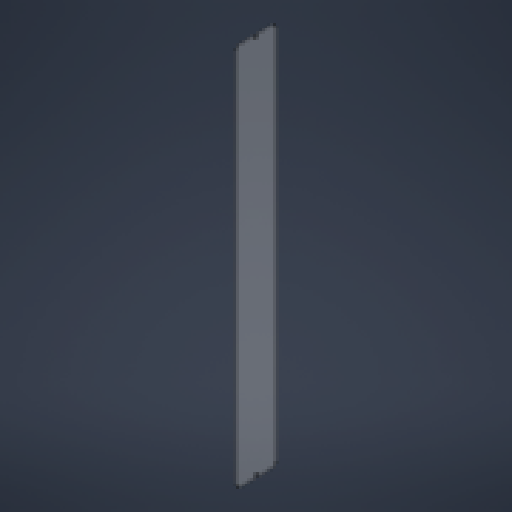
# Autodesk Inventor part: PLATE,BOTTOM,BACK
Saved by Autodesk Inventor 2026 (Build 300175000, 175)
## iProperties
Created: 2026-02-18
Part Number: PLATE,BOTTOM,BACK
Material: Polycarbonate, Clear
Document SubType Name: Modeling
Designer: littl
Density: 1.2 g/cm^3
Appearance: Polycarbonate - Clear
Author: littl
Autodesk Inventor part; units mm, degrees
ref_plane "YZ Plane" through (0, 0, 0) normal (1, 0, 0) x (0, 1, 0)
ref_plane "XZ Plane" through (0, 0, 0) normal (0, 1, 0) x (-1, 0, 0)
ref_plane "XY Plane" through (0, 0, 0) normal (0, 0, 1) x (1, 0, 0)
sketch "Sketch1" plane through (0, 0, 0) normal (1, 0, 0) x (0, 1, 0)
  line L0 (-323.85, -34.925) -> (323.85, -34.925)
  line L1 (323.85, -34.925) -> (323.85, 34.925)
  line L2 (323.85, 34.925) -> (-323.85, 34.925)
  line L3 (-323.85, 34.925) -> (-323.85, -34.925)
  line L4 (-323.85, -34.925) -> (323.85, 34.925) construction
  line L5 (323.85, -34.925) -> (-323.85, 34.925) construction
  line L6 (-323.85, 31.75) -> (-328.6125, 31.75)
  line L7 (-328.6125, 31.75) -> (-328.6125, -31.75)
  line L8 (-328.6125, -31.75) -> (-323.85, -31.75)
  line L9 (-323.85, -31.75) -> (-323.85, 31.75)
  line L10 (323.85, 31.75) -> (328.6125, 31.75)
  line L11 (328.6125, 31.75) -> (328.6125, -31.75)
  line L12 (328.6125, -31.75) -> (323.85, -31.75)
  line L13 (323.85, -31.75) -> (323.85, 31.75)
  line L14 (-328.6125, 3.302) -> (-323.85, 3.302)
  line L15 (-323.85, 3.302) -> (-323.85, -3.302)
  line L16 (-323.85, -3.302) -> (-328.6125, -3.302)
  line L17 (-328.6125, -3.302) -> (-328.6125, 3.302)
  line L18 (323.85, 3.302) -> (328.6125, 3.302)
  line L19 (328.6125, 3.302) -> (328.6125, -3.302)
  line L20 (328.6125, -3.302) -> (323.85, -3.302)
  line L21 (323.85, -3.302) -> (323.85, 3.302)
  point P0 (0, 0)
  point P1 (328.6125, 0)
  point P2 (-328.6125, 0)
  point P3 (-328.6125, 0)
  point P4 (323.85, 0)
  point P5 (323.85, -3.302)
  point P6 (323.85, 3.302)
  point P7 (328.6125, 3.302)
  point P8 (-323.85, 3.302)
  point P9 (-323.85, -3.302)
  point P10 (-328.6125, -3.302)
  dimension "d0" = 69.85
  dimension "d1" = 4.7625
  dimension "d2" = 63.5
  dimension "d3" = 6.604
  dimension "d4" = 6.604
  dimension "d5" = 647.7
  constraints: 44 end point, 10 parallel, 6 midpoint, 6 point on line, 5 horizontal, 5 perpendicular, 4 horizontal alignment, 2 equal length
  measures "d0" distance of L1.end L0.end
  measures "d1" distance of L8.end L7.end
  measures "d2" distance of L7.end L6.end
  measures "d3" distance between parallel lines of L14 L16
  measures "d4" distance between parallel lines of L20 L18
  measures "d5" distance between parallel lines of L1 L9
extrude "Extrusion1" add sketch "Sketch1" along normal blind 3.175 contours L3 L2 L1 L0 | L8 L7 L16 L3 | L1 L20 L11 L12 | L14 L7 L6 L3 | L1 L10 L11 L18
equation "\"d4\" = d3"
body "Solid1"
